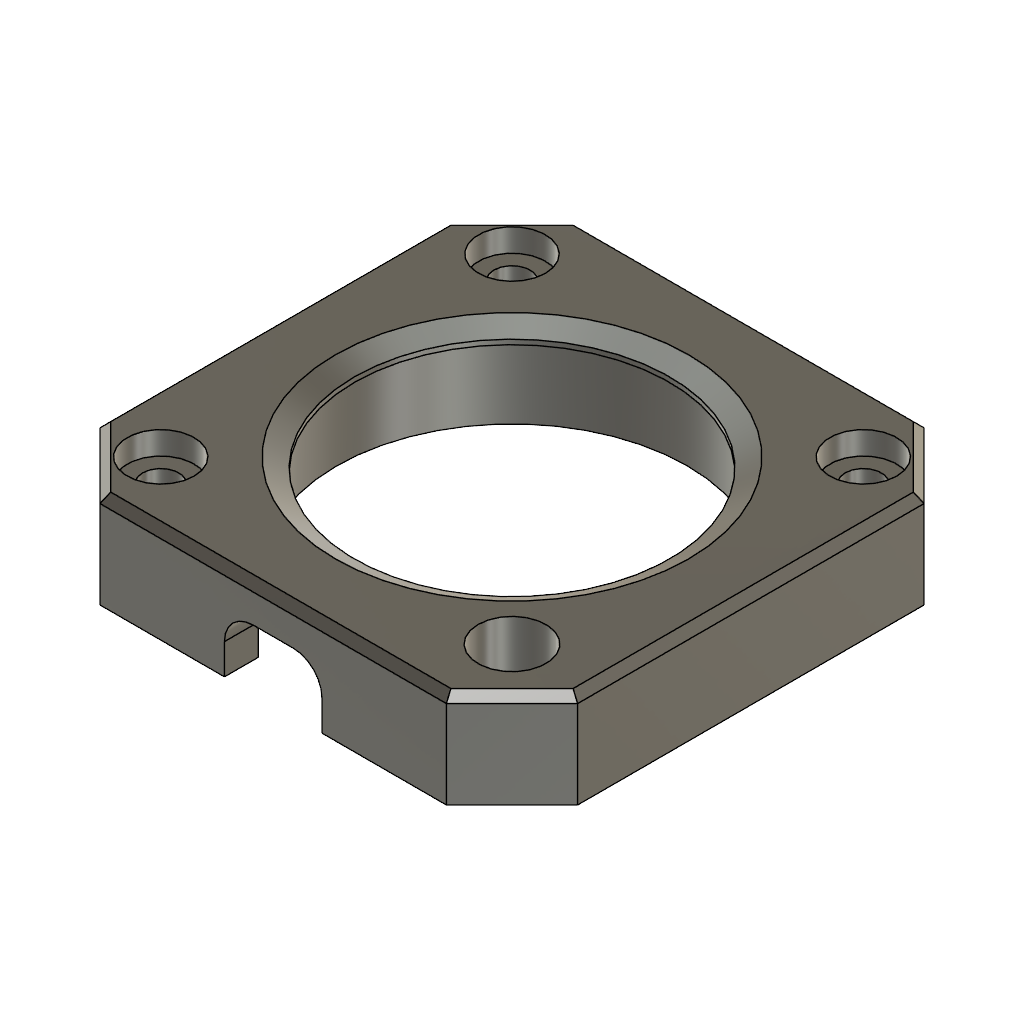
Frontplatte (Autodesk Fusion 360 design; units mm, degrees)
Autodesk Fusion 360 part; units mm, degrees
note: some values were not read from the file. Set by a fixed rule: which face or edge a step refers to.
sketch "Skizze1" plane through (0, 0, 0) normal (0, 0, 1) x (1, 0, 0)
  line L0 (-50, 50) -> (0, 50)
  line L1 (0, 50) -> (0, 0)
  line L2 (0, 0) -> (-50, 0)
  line L3 (-50, 0) -> (-50, 50)
  line L4 (-50, 25) -> (0, 25) construction
  line L5 (-25, 50) -> (-25, 0) construction
  circle A0 centre (-25, 25) radius 16.5
  circle A1 centre (-8.0294, 8.0294) radius 3.55
  line L6 (-50, 50) -> (0, 0) construction
  line L7 (0, 50) -> (-50, 0) construction
  circle A2 centre (-43.3848, 43.3848) radius 1.9
  circle A3 centre (-6.6152, 43.3848) radius 1.9
  circle A4 centre (-43.3848, 6.6152) radius 1.9
  line L8 (-6.8665, 50) -> (0, 43.1335)
  line L9 (-50, 6.8665) -> (-43.1335, 0)
  line L10 (-43.1335, 50) -> (-50, 43.1335)
  line L11 (0, 6.8665) -> (-6.8665, 0)
  line L12 (-8.0294, 16.5147) -> (-16.5147, 8.0294) construction
  line L13 (-16.5147, 8.0294) -> (-8.0294, -0.4558) construction
  line L14 (-8.0294, -0.4558) -> (0.4558, 8.0294) construction
  line L15 (0.4558, 8.0294) -> (-8.0294, 16.5147) construction
  line L16 (-8.0294, 16.5147) -> (-8.0294, -0.4558) construction
  point P0 (-8.0294, 8.0294)
  point P1 (-8.0294, 8.0294)
  dimension "d3" = 33
  dimension "d4" = 7.1
  dimension "d6" = 3.8
  dimension "d7" = 26
  dimension "d8" = 26
  dimension "d9" = 26
  dimension "d42" = 50
  dimension "d43" = 50
  dimension "d44" = 61
  dimension "d45" = 61
  dimension "d46" = 12
  dimension "d47" = 12
  dimension "d54" = 6.5
  constraint horizontal L0
  constraint vertical L1
  constraint horizontal L2
  constraint vertical L3
  constraint coincident L1.end L2.start
  constraint midpoint L3 L4.start
  constraint midpoint L1 L4.end
  constraint midpoint L0 L5.start
  constraint midpoint L2 L5.end
  constraint midpoint L4 A0.centre
  constraint coincident L6 A2.centre
  constraint coincident L7 A3.centre
  constraint coincident L7 A4.centre
  constraint equal A2 A3
  constraint equal A2 A4
  constraint coincident L0 L8.start
  constraint coincident L1 L8.end
  constraint perpendicular L7 L8
  constraint coincident L3 L9.start
  constraint coincident L2 L9.end
  constraint perpendicular L7 L9
  constraint coincident L0 L10.start
  constraint coincident L3 L10.end
  constraint perpendicular L6 L10
  constraint coincident L1 L11.start
  constraint coincident L2 L11.end
  constraint symmetric L6 L8 L9
  constraint symmetric L7 L10 L11
  constraint coincident P1 P0
  constraint parallel L12 L14
  constraint vertical L16
  constraint perpendicular L12 L15
  constraint perpendicular L12 L13
  constraint midpoint L16 P1
  constraint coincident P1 L6
  measures "d3" diameter of A0
  measures "d4" diameter of A1
  measures "d6" diameter of A2
  measures "d7" distance of A0.centre A2.centre
  measures "d8" distance of A0.centre A3.centre
  measures "d9" distance of A0.centre A4.centre
  measures "d42" distance of L0.start L2.end
  measures "d43" distance of L0.start L0.end
  measures "d44" distance of L8 L9
  measures "d45" distance of L10 L11
  measures "d46" distance of L12.start L14.end
  measures "d47" distance of L12.start L12.end
  measures "d54" distance of P1 L11
extrude "Extrusion1" add sketch "Skizze1" along normal blind 3 contours L0 L1 L2 L3 L8 L9 L10 L11
chamfer "Fase1" distance 0.8 angle 45 8 edges at (-25, 0, 3) (-46.5668, 3.4332, 3) (-50, 25, 3) (-46.5668, 46.5668, 3) (-25, 50, 3) (-3.4332, 46.5668, 3) (0, 25, 3) (-3.4332, 3.4332, 3)
chamfer "Fase3" distance 2 distance2 1 1 edges at (-40.3834, 30.9667, 3) measured on face at (-24.589, 46.618, 3)
sketch "Skizze2" plane through (0, 0, 0) normal (0, 0, -1) x (1, 0, 0)
  circle A0 centre (-25, -25) radius 16.5
  circle A1 centre (-43.3848, -43.3848) radius 1.9
  circle A2 centre (-43.3848, -6.6152) radius 1.9
  circle A3 centre (-8.0294, -8.0294) radius 3.55
  circle A4 centre (-6.6152, -43.3848) radius 1.9
  line L0 (-50, -43.1335) -> (-43.1335, -50)
  line L1 (-43.1335, -50) -> (-6.8665, -50)
  line L2 (-6.8665, -50) -> (0, -43.1335)
  line L3 (0, -43.1335) -> (0, -6.8665)
  line L4 (0, -6.8665) -> (-6.8665, 0)
  line L5 (-6.8665, 0) -> (-43.1335, 0)
  line L6 (-43.1335, 0) -> (-50, -6.8665)
  line L7 (-50, -6.8665) -> (-50, -43.1335)
  circle A5 centre (-25, -25) radius 18.35
  line L8 (-14.75, -9.7796) -> (-17.9, -3.55)
  line L9 (-17.9, -3.55) -> (-32.1, -3.55)
  line L10 (-32.1, -3.55) -> (-35.25, -9.7796)
  line L11 (-25, -25) -> (-25, 4.0219) construction
  dimension "d18" = 36.7
  dimension "d19" = 21.45
  dimension "d20" = 20.5
  dimension "d21" = 14.2
  constraint concentric A0 A5
  constraint coincident A5 L8.start
  constraint horizontal L9
  constraint coincident A5 L10.end
  constraint coincident A0.centre A5.centre
  constraint vertical L11
  constraint symmetric L8.end L9.end L11
  constraint symmetric L8.start L10.end L11
  measures "d18" diameter of A5
  measures "d19" distance of A0.centre L9
  measures "d20" distance of L8.start L10.end
  measures "d21" distance of L8.end L9.end
extrude "Extrusion2" cut sketch "Skizze2" against normal blind 1.5 contours A5 | A5 L8 L9 L10
sketch "Skizze3" plane through (0, 0, 0) normal (0, -1, 0) x (1, 0, 0)
  line L0 (-6.8665, 2.2) -> (-43.1335, 2.2)
  line L1 (-43.1335, 2.2) -> (-43.1335, 0)
  line L2 (-43.1335, 0) -> (-6.8665, 0)
  line L3 (-6.8665, 0) -> (-6.8665, 2.2)
  line L4 (-41.5, 1.5) -> (-8.5, 1.5)
  line L5 (-41.5, 2) -> (-8.5, 2)
  line L6 (-25, 1.5) -> (-25, -10) construction
  line L7 (-22.9, -6.8) -> (-27.1, -6.8)
  line L8 (-22.9, -0.8) -> (-27.1, -0.8)
  arc A0 (-27.1, -0.8) -> (-27.1, -6.8) centre (-27.1, -3.8) ccw
  arc A1 (-22.9, -6.8) -> (-22.9, -0.8) centre (-22.9, -3.8) ccw
  line L9 (-19.9, -3.8) -> (-30.1, -3.8) construction
  line L10 (-25, -5.5) -> (-25, -2.1) construction
  line L11 (-22.9, -6.8) -> (-19.9, -6.8)
  line L12 (-19.9, -6.8) -> (-19.9, -3.8)
  line L13 (-27.1, -6.8) -> (-30.1, -6.8)
  line L14 (-30.1, -6.8) -> (-30.1, -3.8)
  line L15 (-30.1, -6.8) -> (-19.9, -6.8)
  line L16 (-19.9, -6.8) -> (-19.9, -8.8)
  line L17 (-19.9, -8.8) -> (-30.1, -8.8)
  line L18 (-30.1, -8.8) -> (-30.1, -6.8)
  point P0 (-25, -2.1)
  point P1 (-25, -5.5)
  point P2 (-25, -3.8)
  point P3 (-25, -3.8)
  dimension "d24" = 3.6
  dimension "d25" = 7
  dimension "d27" = 6
  dimension "d31" = 10.2
  dimension "d53" = 2
  constraint midpoint L4 L6.start
  constraint perpendicular L2 L6
  constraint coincident L6 P0
  constraint coincident L6 P1
  constraint horizontal L7
  constraint horizontal L8
  constraint tangent L7 A1
  constraint tangent L7 A0
  constraint tangent L8 A0
  constraint tangent L8 A1
  constraint symmetric L6 A1.centre A0.centre
  constraint coincident A1 L9.start
  constraint midpoint A0 L9.end
  constraint horizontal L9
  constraint coincident P1 L10.start
  constraint coincident P0 L10.end
  constraint midpoint L10 P3
  constraint midpoint L9 P3
  constraint coincident P3 P2
  constraint parallel L7 L11
  constraint perpendicular L7 L12
  constraint horizontal L13
  constraint perpendicular L13 L14
  constraint coincident L7.start A1.start
  constraint coincident L7.end A0.end
  constraint coincident L9.start L12.end
  constraint coincident L9.end L14.end
  constraint horizontal L15
  constraint vertical L16
  constraint horizontal L17
  constraint vertical L18
  constraint coincident L11.end L12.start
  measures "d24" distance of L6.start P0
  measures "d25" distance of L6.start P1
  measures "d27" distance of L7 L8
  measures "d31" distance of L9.start L9.end
  measures "d53" distance of L13.end L17.end
extrude "Extrusion3" add 1 faces at (-47.7677, 25.4366, 0) along direction (0, 0, -1) blind 7
extrude "Extrusion4" cut sketch "Skizze3" against normal up to surface (3.55 mm away) contours L7 L11 L13 L15 L16 L17 L18 | L7 L8 A0 A1 L15 | A1 L11 L12 L15 | A0 L13 L14 L15
sketch "Skizze4" plane through (0, 0, -7) normal (0, 0, -1) x (1, 0, 0)
  circle A0 centre (-43.3848, -43.3848) radius 1.9
  circle A1 centre (-6.6152, -43.3848) radius 1.9
  arc A2 (-35.25, -9.7796) -> (-14.75, -9.7796) centre (-25, -25) ccw
  arc A3 (-35.25, -9.7796) -> (-14.75, -9.7796) centre (-25, -25) ccw
  circle A4 centre (-8.0294, -8.0294) radius 3.55
  circle A5 centre (-8.0294, -8.0294) radius 3.55
  circle A6 centre (-43.3848, -6.6152) radius 1.9
  circle A7 centre (-8.0294, -8.0294) radius 3.5
  circle A8 centre (-8.0294, -8.0294) radius 5
  circle A9 centre (-6.6152, -43.3848) radius 1.1
  circle A10 centre (-6.6152, -43.3848) radius 3
  circle A11 centre (-43.3848, -43.3848) radius 1.1
  circle A12 centre (-43.3848, -43.3848) radius 3
  circle A13 centre (-43.3848, -6.6152) radius 1.1
  circle A14 centre (-43.3848, -6.6152) radius 3
  circle A15 centre (-43.3848, -43.3848) radius 1.9
  circle A16 centre (-6.6152, -43.3848) radius 1.9
  circle A17 centre (-43.3848, -6.6152) radius 1.9
  dimension "d49" = 6
  dimension "d50" = 10
  constraint concentric A4 A7
  constraint concentric A7 A8
  constraint concentric A1 A9
  constraint concentric A1 A10
  constraint concentric A0 A11
  constraint concentric A0 A12
  constraint concentric A6 A13
  constraint concentric A6 A14
  constraint equal A12 A14
  constraint equal A10 A12
  measures "d49" diameter of A14
  measures "d50" diameter of A8
extrude "Extrusion5" cut sketch "Skizze4" against normal blind 4 contours A10 | A12 | A14
extrude "Extrusion6" cut sketch "Skizze4" against normal blind 3 contours A8
sketch "Skizze5" plane through (0, 0, 3) normal (0, 0, 1) x (-1, 0, 0)
  line L0 (7.1979, -49.2) -> (42.8021, -49.2)
  line L1 (42.8021, -49.2) -> (49.2, -42.8021)
  line L2 (49.2, -42.8021) -> (49.2, -7.1979)
  line L3 (49.2, -7.1979) -> (42.8021, -0.8)
  line L4 (42.8021, -0.8) -> (7.1979, -0.8)
  line L5 (7.1979, -0.8) -> (0.8, -7.1979)
  line L6 (0.8, -7.1979) -> (0.8, -42.8021)
  line L7 (0.8, -42.8021) -> (7.1979, -49.2)
  circle A0 centre (43.3848, -43.3848) radius 1.9
  circle A1 centre (43.3848, -6.6152) radius 1.9
  circle A2 centre (6.6152, -43.3848) radius 1.9
  circle A3 centre (8.0294, -8.0294) radius 3.55
  circle A4 centre (25, -25) radius 18.5
  circle A5 centre (6.6152, -43.3848) radius 1.9
  circle A6 centre (6.6152, -43.3848) radius 1.9
  circle A7 centre (43.3848, -43.3848) radius 1.9
  circle A8 centre (43.3848, -43.3848) radius 1.9
  circle A9 centre (43.3848, -6.6152) radius 1.9
  circle A10 centre (43.3848, -6.6152) radius 1.9
  circle A11 centre (43.3848, -43.3848) radius 3.5
  circle A12 centre (43.3848, -6.6152) radius 3.5
  circle A13 centre (6.6152, -43.3848) radius 3.5
  dimension "d55" = 7
  constraint concentric A7 A11
  constraint concentric A9 A12
  constraint concentric A5 A13
  constraint equal A11 A13
  constraint equal A11 A12
  measures "d55" diameter of A11
extrude "Extrusion7" cut sketch "Skizze5" against normal blind 2.4 contours A11 | A12 | A13
sketch "Skizze6" plane through (0, 0, -7) normal (0, 0, -1) x (1, 0, 0)
  circle A0 centre (-8.0294, -8.0294) radius 5
  line L0 (-30.1, -3.55) -> (-30.1, 0)
  line L1 (-30.1, 0) -> (-43.1335, 0)
  line L2 (-43.1335, 0) -> (-50, -6.8665)
  line L3 (-50, -6.8665) -> (-50, -43.1335)
  line L4 (-50, -43.1335) -> (-43.1335, -50)
  line L5 (-43.1335, -50) -> (-6.8665, -50)
  line L6 (-6.8665, -50) -> (0, -43.1335)
  line L7 (0, -43.1335) -> (0, -6.8665)
  line L8 (0, -6.8665) -> (-6.8665, 0)
  line L9 (-6.8665, 0) -> (-19.9, 0)
  line L10 (-19.9, 0) -> (-19.9, -3.55)
  line L11 (-19.9, -3.55) -> (-17.9, -3.55)
  line L12 (-17.9, -3.55) -> (-14.75, -9.7796)
  arc A1 (-35.25, -9.7796) -> (-14.75, -9.7796) centre (-25, -25) ccw
  line L13 (-35.25, -9.7796) -> (-32.1, -3.55)
  line L14 (-32.1, -3.55) -> (-30.1, -3.55)
  circle A2 centre (-6.6152, -43.3848) radius 3
  circle A3 centre (-43.3848, -43.3848) radius 3
  circle A4 centre (-43.3848, -6.6152) radius 3
  circle A5 centre (-6.6152, -43.3848) radius 3
  circle A6 centre (-43.3848, -43.3848) radius 3
  circle A7 centre (-43.3848, -6.6152) radius 3
  circle A8 centre (-8.0294, -8.0294) radius 5
  circle A9 centre (-25, -25) radius 19.5
  dimension "d58" = 39
  constraint concentric A2 A5
  constraint concentric A3 A6
  constraint concentric A4 A7
  constraint concentric A0 A8
  constraint concentric A1 A9
  measures "d58" diameter of A9
equation "d8 = d7"
equation "d9 = d7"
equation "d54 = 6.85 mm - 0.35 mm"
